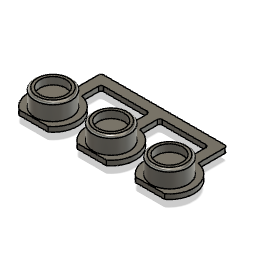
VFD_NTP_CLOCK_BUTTON_V2.2 v2 (Autodesk Fusion 360 design; units mm, degrees)
Autodesk Fusion 360 part; units mm, degrees
sketch "スケッチ1" plane through (0, 0, 0) normal (0, 1, 0) x (1, 0, 0)
  circle A0 centre (0, 0) radius 5
  circle A1 centre (12, 0) radius 5
  circle A2 centre (-12, 0) radius 5
  line L0 (-13.0007, 4.8988) -> (-13.0007, 10.8988)
  line L1 (-10.9848, 4.8958) -> (-10.9848, 8.8958)
  line L2 (-13.0007, 10.8988) -> (12.9993, 10.8988)
  line L3 (12.9993, 10.8988) -> (12.9993, 4.8991)
  line L4 (11.0007, 4.8991) -> (11.0007, 9)
  line L5 (11.0007, 9) -> (1, 9)
  line L6 (1, 9) -> (1, 4.899)
  line L7 (-10.9848, 8.8958) -> (-1, 8.8958)
  line L8 (-1, 8.8958) -> (-1, 4.899)
  dimension "d1" = 10
  dimension "d2" = 10
  dimension "d3" = 6
  dimension "d4" = 4
  dimension "d5" = 26
  constraint coincident A0.centre origin
  constraint coincident A2 L0.start
  constraint vertical L0
  constraint coincident A2 L1.start
  constraint parallel L0 L1
  constraint perpendicular L0 L2
  constraint coincident A1 L3.end
  constraint perpendicular L2 L3
  constraint coincident A1 L4.start
  constraint perpendicular L2 L4
  constraint perpendicular L4 L5
  constraint coincident A0 L6.end
  constraint perpendicular L5 L6
  constraint perpendicular L1 L7
  constraint coincident A0 L8.end
  constraint perpendicular L7 L8
  measures "d1" diameter of A0
  measures "d2" diameter of A1
  measures "d3" distance of L0.start L0.end
  measures "d4" distance of L1.start L1.end
  measures "d5" distance of L0.end L2.end
extrude "押し出し1" add sketch "スケッチ1" along normal blind 1
sketch "スケッチ2" plane through (0, 1, 0) normal (0, 1, 0) x (-1, 0, 0)
  arc A0 (13.0007, -4.8988) -> (10.9848, -4.8958) centre (12, 0) ccw
  line L0 (10.9848, -4.8958) -> (10.9848, -8.8958)
  line L1 (10.9848, -8.8958) -> (1, -8.8958)
  line L2 (1, -8.8958) -> (1, -4.899)
  arc A1 (1, -4.899) -> (-1, -4.899) centre (0, 0) ccw
  line L3 (-1, -4.899) -> (-1, -9)
  line L4 (-1, -9) -> (-11.0007, -9)
  line L5 (-11.0007, -9) -> (-11.0007, -4.8991)
  arc A2 (-11.0007, -4.8991) -> (-12.9993, -4.8991) centre (-12, 0) ccw
  line L6 (-12.9993, -4.8991) -> (-12.9993, -10.8988)
  line L7 (-12.9993, -10.8988) -> (13.0007, -10.8988)
  line L8 (13.0007, -10.8988) -> (13.0007, -4.8988)
  circle A3 centre (0, 0) radius 3.75
  circle A4 centre (12, 0) radius 3.75
  circle A5 centre (-12, 0) radius 3.75
  dimension "d8" = 7.5
  dimension "d9" = 7.5
  dimension "d10" = 7.5
  constraint concentric A1 A3
  constraint concentric A0 A4
  constraint concentric A2 A5
  measures "d8" diameter of A3
  measures "d9" diameter of A4
  measures "d10" diameter of A5
extrude "押し出し2" add sketch "スケッチ2" along normal blind 3.5 contours A3 | A4 | A5
sketch "スケッチ3" plane through (0, 4.5, 0) normal (0, 1, 0) x (-1, 0, 0)
  circle A0 centre (12, 0) radius 3.75
  circle A1 centre (12, 0) radius 2.7
  circle A2 centre (0, 0) radius 2.7
  circle A3 centre (-12, 0) radius 2.7
  dimension "d13" = 5.4
  dimension "d14" = 5.4
  dimension "d15" = 5.4
  constraint concentric A0 A1
  constraint coincident A2.centre origin
  measures "d13" diameter of A1
  measures "d14" diameter of A2
  measures "d15" diameter of A3
extrude "押し出し3" cut sketch "スケッチ3" against normal blind 1.5 contours A1 | A2 | A3
fillet "フィレット1" radius 0.5 1 edges at (1, 0.5, -9)
fillet "フィレット2" radius 0.5 1 edges at (11.0007, 0.5, -9)
fillet "フィレット3" radius 0.5 1 edges at (-1, 0.5, -8.8958)
fillet "フィレット4" radius 0.5 1 edges at (-10.9848, 0.5, -8.8958)
fillet "フィレット5" radius 0.5 1 edges at (12.9993, 0.5, -10.8988)
fillet "フィレット6" radius 0.5 1 edges at (-13.0007, 0.5, -10.8988)
fillet "フィレット7" radius 0.5 3 edges at (15.4962, 4.5, -1.3561) (3.4962, 4.5, -1.3561) (-8.5038, 4.5, -1.3561)
sketch "スケッチ4" plane through (0, 0, 0) normal (0, -1, 0) x (1, 0, 0)
  arc A0 (-13.0007, -10.3988) -> (-12.5007, -10.8988) centre (-12.5007, -10.3988) ccw
  line L0 (-12.5007, -10.8988) -> (12.4993, -10.8988)
  arc A1 (12.4993, -10.8988) -> (12.9993, -10.3988) centre (12.4993, -10.3988) ccw
  line L1 (12.9993, -10.3988) -> (12.9993, -4.8991)
  arc A2 (12.9993, -4.8991) -> (11.0007, -4.8991) centre (12, 0) ccw
  line L2 (11.0007, -4.8991) -> (11.0007, -8.5)
  arc A3 (10.5007, -9) -> (11.0007, -8.5) centre (10.5007, -8.5) ccw
  line L3 (10.5007, -9) -> (1.5, -9)
  arc A4 (1, -8.5) -> (1.5, -9) centre (1.5, -8.5) ccw
  line L4 (1, -8.5) -> (1, -4.899)
  arc A5 (1, -4.899) -> (-1, -4.899) centre (0, 0) ccw
  line L5 (-1, -4.899) -> (-1, -8.3958)
  arc A6 (-1.5, -8.8958) -> (-1, -8.3958) centre (-1.5, -8.3958) ccw
  line L6 (-1.5, -8.8958) -> (-10.4848, -8.8958)
  arc A7 (-10.9848, -8.3958) -> (-10.4848, -8.8958) centre (-10.4848, -8.3958) ccw
  line L7 (-10.9848, -8.3958) -> (-10.9848, -4.8958)
  arc A8 (-10.9848, -4.8958) -> (-13.0007, -4.8988) centre (-12, 0) ccw
  line L8 (-13.0007, -4.8988) -> (-13.0007, -10.3988)
  circle A9 centre (-12, 0) radius 2
  circle A10 centre (0, 0) radius 2
  circle A11 centre (12, 0) radius 2
  dimension "d32" = 4
  constraint concentric A8 A9
  constraint concentric A5 A10
  constraint concentric A2 A11
  measures "d32" diameter of A9
extrude "押し出し4" add sketch "スケッチ4" along normal blind 1.5 contours A9 | A10 | A11
fillet "フィレット8" radius 0.5 3 edges at (-13.8647, -1.5, -0.7232) (-1.8647, -1.5, -0.7232) (10.1353, -1.5, -0.7232)
sketch "スケッチ5" plane through (0, 1, 0) normal (0, 1, 0) x (-1, 0, 0)
  arc A0 (12.5007, -10.8988) -> (13.0007, -10.3988) centre (12.5007, -10.3988) ccw
  line L0 (13.0007, -10.3988) -> (13.0007, -4.8988)
  arc A1 (13.0007, -4.8988) -> (10.9848, -4.8958) centre (12, 0) ccw
  line L1 (10.9848, -4.8958) -> (10.9848, -8.3958)
  arc A2 (10.4848, -8.8958) -> (10.9848, -8.3958) centre (10.4848, -8.3958) ccw
  line L2 (10.4848, -8.8958) -> (1.5, -8.8958)
  arc A3 (1, -8.3958) -> (1.5, -8.8958) centre (1.5, -8.3958) ccw
  line L3 (1, -8.3958) -> (1, -4.899)
  arc A4 (1, -4.899) -> (-1, -4.899) centre (0, 0) ccw
  line L4 (-1, -4.899) -> (-1, -8.5)
  arc A5 (-1.5, -9) -> (-1, -8.5) centre (-1.5, -8.5) ccw
  line L5 (-1.5, -9) -> (-10.5007, -9)
  arc A6 (-11.0007, -8.5) -> (-10.5007, -9) centre (-10.5007, -8.5) ccw
  line L6 (-11.0007, -8.5) -> (-11.0007, -4.8991)
  arc A7 (-11.0007, -4.8991) -> (-12.9993, -4.8991) centre (-12, 0) ccw
  line L7 (-12.9993, -4.8991) -> (-12.9993, -10.3988)
  arc A8 (-12.9993, -10.3988) -> (-12.4993, -10.8988) centre (-12.4993, -10.3988) ccw
  line L8 (-12.4993, -10.8988) -> (12.5007, -10.8988)
  circle A9 centre (-12, 0) radius 3.75
  circle A10 centre (0, 0) radius 3.75
  circle A11 centre (12, 0) radius 3.75
  line L9 (17, 5.5) -> (-17, 5.5)
  line L10 (-17, 5.5) -> (-17, 4)
  line L11 (-17, 4) -> (17, 4)
  line L12 (17, 4) -> (17, 5.5)
  constraint horizontal L9
  constraint vertical L10
  constraint horizontal L11
  constraint vertical L12
extrude "押し出し5" cut sketch "スケッチ5" against normal blind 1 contours A1 L11 | A7 L11 | A4 L11
